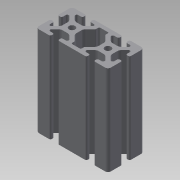
# Autodesk Inventor part: 40-4080
Saved by Autodesk Inventor 2013 (Build 170138000, 138)
## iProperties
Created: 2014-04-23
Part Number: 40-4080
Material: Generic
Document SubType Name: Modeling
Designer: Ross Bowman
Density: 1 g/cm^3
Engineer: Ross Bowman
Catalog Web Link: 8020.net
Vendor: 80/20 Inc.
Company: 80/20 Inc.
Author: Ross Bowman
Keywords: 80/20 , 8020 , T-Slot , Extrusion
Material: 6105-T5 Aluminum
Autodesk Inventor part; units mm, degrees
ref_plane "YZ Plane" through (0, 0, 0) normal (1, 0, 0) x (0, 1, 0)
ref_plane "XZ Plane" through (0, 0, 0) normal (0, 1, 0) x (-1, 0, 0)
ref_plane "XY Plane" through (0, 0, 0) normal (0, 0, 1) x (1, 0, 0)
sketch "Sketch1" plane through (0, 0, 0) normal (0, 0, 1) x (1, 0, 0)
  circle A0 centre (20, 0) radius 3.4
  line L0 (-11.2012, -5.7441) -> (-5.7137, -11.2316)
  arc A1 (-12.2841, -2.725) -> (-11.2012, -5.7441) centre (-7.5341, -2.725) ccw
  line L1 (-12.2841, 3.2591) -> (-12.2841, -2.725)
  arc A2 (-10.5988, 6.3465) -> (-12.2841, 3.2591) centre (-7.5685, 2.6887) ccw
  line L2 (-5.7137, 11.2316) -> (-10.5988, 6.3465)
  arc A3 (-5.7137, 11.2316) -> (-5.3418, 12.1296) centre (-6.6118, 12.1296) ccw
  line L3 (-5.3418, 14.41) -> (-5.3418, 12.1296)
  arc A4 (-4.0718, 15.68) -> (-5.3418, 14.41) centre (-4.0718, 14.41) ccw
  line L4 (4.0718, 15.68) -> (-4.0718, 15.68)
  arc A5 (5.3418, 14.41) -> (4.0718, 15.68) centre (4.0718, 14.41) ccw
  line L5 (5.3418, 12.1296) -> (5.3418, 14.41)
  arc A6 (5.3418, 12.1296) -> (5.7137, 11.2316) centre (6.6118, 12.1296) ccw
  line L6 (10.5988, 6.3465) -> (5.7137, 11.2316)
  arc A7 (12.2841, 3.2591) -> (10.5988, 6.3465) centre (7.5685, 2.6887) ccw
  line L7 (12.2841, -2.725) -> (12.2841, 3.2591)
  arc A8 (11.2012, -5.7441) -> (12.2841, -2.725) centre (7.5341, -2.725) ccw
  line L8 (5.7137, -11.2316) -> (11.2012, -5.7441)
  arc A9 (5.7137, -11.2316) -> (5.3418, -12.1296) centre (6.6118, -12.1296) ccw
  line L9 (5.3418, -14.41) -> (5.3418, -12.1296)
  arc A10 (4.0718, -15.68) -> (5.3418, -14.41) centre (4.0718, -14.41) ccw
  line L10 (-4.0718, -15.68) -> (4.0718, -15.68)
  arc A11 (-5.3418, -14.41) -> (-4.0718, -15.68) centre (-4.0718, -14.41) ccw
  line L11 (-5.3418, -12.1296) -> (-5.3418, -14.41)
  arc A12 (-5.3418, -12.1296) -> (-5.7137, -11.2316) centre (-6.6118, -12.1296) ccw
  circle A13 centre (-20, 0) radius 3.4
  arc A14 (14.37, -20) -> (15.94, -18.43) centre (14.37, -18.43) ccw
  line L12 (15.94, -18.43) -> (15.94, -17.25)
  arc A15 (15.94, -17.25) -> (14.37, -15.68) centre (14.37, -17.25) ccw
  line L13 (14.37, -15.68) -> (11.285, -15.68)
  arc A16 (9.715, -14.11) -> (11.285, -15.68) centre (11.285, -14.11) ccw
  line L14 (9.715, -14.11) -> (9.715, -13.6545)
  arc A17 (9.9376, -13.1171) -> (9.715, -13.6545) centre (10.475, -13.6545) ccw
  line L15 (9.9376, -13.1171) -> (13.6905, -9.3642)
  arc A18 (16.6585, -7.7) -> (13.6905, -9.3642) centre (17.3435, -12.4003) ccw
  line L16 (16.6585, -7.7) -> (23.3415, -7.7)
  arc A19 (26.3095, -9.3642) -> (23.3415, -7.7) centre (22.6565, -12.4003) ccw
  line L17 (26.3095, -9.3642) -> (30.0624, -13.1171)
  arc A20 (30.285, -13.6545) -> (30.0624, -13.1171) centre (29.525, -13.6545) ccw
  line L18 (30.285, -13.6545) -> (30.285, -14.11)
  arc A21 (28.715, -15.68) -> (30.285, -14.11) centre (28.715, -14.11) ccw
  line L19 (28.715, -15.68) -> (25.63, -15.68)
  arc A22 (25.63, -15.68) -> (24.06, -17.25) centre (25.63, -17.25) ccw
  line L20 (24.06, -17.25) -> (24.06, -18.4389)
  arc A23 (24.06, -18.4389) -> (25.797, -20) centre (25.63, -18.4389) ccw
  line L21 (25.797, -20) -> (37.0574, -20)
  arc A24 (37.0574, -20) -> (40, -16.83) centre (36.83, -16.8382) ccw
  line L22 (40, -16.83) -> (40, -5.5696)
  arc A25 (40, -5.5696) -> (38.4312, -4.06) centre (38.4312, -5.63) ccw
  line L23 (38.4312, -4.06) -> (37.25, -4.06)
  arc A26 (37.25, -4.06) -> (35.68, -5.63) centre (37.25, -5.63) ccw
  line L24 (35.68, -5.63) -> (35.68, -8.715)
  arc A27 (34.111, -10.3398) -> (35.68, -8.715) centre (34.111, -8.7698) ccw
  line L25 (34.111, -10.3398) -> (33.7093, -10.3398)
  arc A28 (33.1719, -10.1172) -> (33.7093, -10.3398) centre (33.7093, -9.5798) ccw
  line L26 (33.1719, -10.1172) -> (28.9155, -5.8608)
  arc A29 (27.7159, -2.502) -> (28.9155, -5.8608) centre (32.4617, -2.7006) ccw
  line L27 (27.7159, -2.502) -> (27.7159, 2.571)
  arc A30 (29.0111, 5.9564) -> (27.7159, 2.571) centre (32.4643, 2.6948) ccw
  line L28 (29.0111, 5.9564) -> (33.1135, 10.0588)
  arc A31 (33.6509, 10.2814) -> (33.1135, 10.0588) centre (33.6509, 9.5214) ccw
  line L29 (33.6509, 10.2814) -> (34.11, 10.2814)
  arc A32 (35.68, 8.7114) -> (34.11, 10.2814) centre (34.11, 8.7114) ccw
  line L30 (35.68, 8.7114) -> (35.68, 5.6264)
  arc A33 (35.68, 5.6264) -> (37.1443, 4.06) centre (37.25, 5.6264) ccw
  line L31 (37.1443, 4.06) -> (38.3243, 4.06)
  arc A34 (38.3243, 4.06) -> (40, 5.5825) centre (38.4306, 5.6264) ccw
  line L32 (40, 5.5825) -> (40, 16.8406)
  arc A35 (40, 16.8406) -> (36.83, 20) centre (36.83, 16.83) ccw
  line L33 (36.83, 20) -> (25.5696, 20)
  arc A36 (25.5696, 20) -> (24.06, 18.4312) centre (25.63, 18.4312) ccw
  line L34 (24.06, 18.4312) -> (24.06, 17.25)
  arc A37 (24.06, 17.25) -> (25.63, 15.68) centre (25.63, 17.25) ccw
  line L35 (25.63, 15.68) -> (28.715, 15.68)
  arc A38 (30.285, 14.11) -> (28.715, 15.68) centre (28.715, 14.11) ccw
  line L36 (30.285, 14.11) -> (30.285, 13.6545)
  arc A39 (30.0624, 13.1171) -> (30.285, 13.6545) centre (29.525, 13.6545) ccw
  line L37 (30.0624, 13.1171) -> (25.9081, 8.9628)
  arc A40 (22.5494, 7.7) -> (25.9081, 8.9628) centre (22.6809, 12.4482) ccw
  line L38 (22.5494, 7.7) -> (17.4506, 7.7)
  arc A41 (14.0919, 8.9628) -> (17.4506, 7.7) centre (17.3191, 12.4482) ccw
  line L39 (14.0919, 8.9628) -> (9.9376, 13.1171)
  arc A42 (9.715, 13.6545) -> (9.9376, 13.1171) centre (10.475, 13.6545) ccw
  line L40 (9.715, 13.6545) -> (9.715, 14.11)
  arc A43 (11.285, 15.68) -> (9.715, 14.11) centre (11.285, 14.11) ccw
  line L41 (11.285, 15.68) -> (14.37, 15.68)
  arc A44 (14.37, 15.68) -> (15.94, 17.1729) centre (14.3719, 17.25) ccw
  line L42 (15.94, 17.1729) -> (15.94, 18.3529)
  arc A45 (15.94, 18.3529) -> (14.3719, 20) centre (14.3719, 18.43) ccw
  line L43 (14.3719, 20) -> (-14.3719, 20)
  arc A46 (-14.3719, 20) -> (-15.94, 18.3529) centre (-14.3719, 18.43) ccw
  line L44 (-15.94, 18.3529) -> (-15.94, 17.1729)
  arc A47 (-15.94, 17.1729) -> (-14.37, 15.68) centre (-14.3719, 17.25) ccw
  line L45 (-14.37, 15.68) -> (-11.285, 15.68)
  arc A48 (-9.715, 14.11) -> (-11.285, 15.68) centre (-11.285, 14.11) ccw
  line L46 (-9.715, 14.11) -> (-9.715, 13.6545)
  arc A49 (-9.9376, 13.1171) -> (-9.715, 13.6545) centre (-10.475, 13.6545) ccw
  line L47 (-9.9376, 13.1171) -> (-14.0919, 8.9628)
  arc A50 (-17.4506, 7.7) -> (-14.0919, 8.9628) centre (-17.3191, 12.4482) ccw
  line L48 (-17.4506, 7.7) -> (-22.5494, 7.7)
  arc A51 (-25.9081, 8.9628) -> (-22.5494, 7.7) centre (-22.6809, 12.4482) ccw
  line L49 (-25.9081, 8.9628) -> (-30.0624, 13.1171)
  arc A52 (-30.285, 13.6545) -> (-30.0624, 13.1171) centre (-29.525, 13.6545) ccw
  line L50 (-30.285, 13.6545) -> (-30.285, 14.11)
  arc A53 (-28.715, 15.68) -> (-30.285, 14.11) centre (-28.715, 14.11) ccw
  line L51 (-28.715, 15.68) -> (-25.63, 15.68)
  arc A54 (-25.63, 15.68) -> (-24.06, 17.25) centre (-25.63, 17.25) ccw
  line L52 (-24.06, 17.25) -> (-24.06, 18.4312)
  arc A55 (-24.06, 18.4312) -> (-25.5696, 20) centre (-25.63, 18.4312) ccw
  line L53 (-25.5696, 20) -> (-36.83, 20)
  arc A56 (-36.83, 20) -> (-40, 16.8406) centre (-36.83, 16.83) ccw
  line L54 (-40, 16.8406) -> (-40, 5.5825)
  arc A57 (-40, 5.5825) -> (-38.3243, 4.06) centre (-38.4306, 5.6264) ccw
  line L55 (-38.3243, 4.06) -> (-37.1443, 4.06)
  arc A58 (-37.1443, 4.06) -> (-35.68, 5.6264) centre (-37.25, 5.6264) ccw
  line L56 (-35.68, 5.6264) -> (-35.68, 8.7114)
  arc A59 (-34.11, 10.2814) -> (-35.68, 8.7114) centre (-34.11, 8.7114) ccw
  line L57 (-34.11, 10.2814) -> (-33.6509, 10.2814)
  arc A60 (-33.1135, 10.0588) -> (-33.6509, 10.2814) centre (-33.6509, 9.5214) ccw
  line L58 (-33.1135, 10.0588) -> (-29.0111, 5.9564)
  arc A61 (-27.7159, 2.571) -> (-29.0111, 5.9564) centre (-32.4643, 2.6948) ccw
  line L59 (-27.7159, 2.571) -> (-27.7159, -2.502)
  arc A62 (-28.9155, -5.8608) -> (-27.7159, -2.502) centre (-32.4617, -2.7006) ccw
  line L60 (-28.9155, -5.8608) -> (-33.1719, -10.1172)
  arc A63 (-33.7093, -10.3398) -> (-33.1719, -10.1172) centre (-33.7093, -9.5798) ccw
  line L61 (-33.7093, -10.3398) -> (-34.111, -10.3398)
  arc A64 (-35.68, -8.715) -> (-34.111, -10.3398) centre (-34.111, -8.7698) ccw
  line L62 (-35.68, -8.715) -> (-35.68, -5.63)
  arc A65 (-35.68, -5.63) -> (-37.25, -4.06) centre (-37.25, -5.63) ccw
  line L63 (-37.25, -4.06) -> (-38.4312, -4.06)
  arc A66 (-38.4312, -4.06) -> (-40, -5.5696) centre (-38.4312, -5.63) ccw
  line L64 (-40, -5.5696) -> (-40, -16.83)
  arc A67 (-40, -16.83) -> (-37.0574, -20) centre (-36.83, -16.8382) ccw
  line L65 (-37.0574, -20) -> (-25.797, -20)
  arc A68 (-25.797, -20) -> (-24.06, -18.4389) centre (-25.63, -18.4389) ccw
  line L66 (-24.06, -18.4389) -> (-24.06, -17.25)
  arc A69 (-24.06, -17.25) -> (-25.63, -15.68) centre (-25.63, -17.25) ccw
  line L67 (-25.63, -15.68) -> (-28.715, -15.68)
  arc A70 (-30.285, -14.11) -> (-28.715, -15.68) centre (-28.715, -14.11) ccw
  line L68 (-30.285, -14.11) -> (-30.285, -13.6545)
  arc A71 (-30.0624, -13.1171) -> (-30.285, -13.6545) centre (-29.525, -13.6545) ccw
  line L69 (-30.0624, -13.1171) -> (-26.3095, -9.3642)
  arc A72 (-23.3415, -7.7) -> (-26.3095, -9.3642) centre (-22.6565, -12.4003) ccw
  line L70 (-23.3415, -7.7) -> (-16.6585, -7.7)
  arc A73 (-13.6905, -9.3642) -> (-16.6585, -7.7) centre (-17.3435, -12.4003) ccw
  line L71 (-13.6905, -9.3642) -> (-9.9376, -13.1171)
  arc A74 (-9.715, -13.6545) -> (-9.9376, -13.1171) centre (-10.475, -13.6545) ccw
  line L72 (-9.715, -13.6545) -> (-9.715, -14.11)
  arc A75 (-11.285, -15.68) -> (-9.715, -14.11) centre (-11.285, -14.11) ccw
  line L73 (-11.285, -15.68) -> (-14.37, -15.68)
  arc A76 (-14.37, -15.68) -> (-15.94, -17.25) centre (-14.37, -17.25) ccw
  line L74 (-15.94, -17.25) -> (-15.94, -18.43)
  arc A77 (-15.94, -18.43) -> (-14.37, -20) centre (-14.37, -18.43) ccw
  line L75 (-14.37, -20) -> (14.37, -20)
  point P0 (0, 0)
  constraints: 152 end point, 152 point on circle, 78 centre point
extrude "Extrusion1" add sketch "Sketch1" against normal blind 100
body "Solid1"
